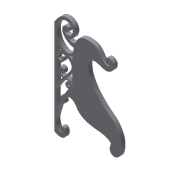
# Autodesk Inventor part: Sleigh
Saved by Autodesk Inventor 2014 (Build 180170000, 170)
## iProperties
Created: 2014-01-28
Part Number: Sleigh
Material: Generic
Document SubType Name: Modeling
Designer: caovt
Mass: 48.764 g
Surface Area: 236.408 cm^2
Volume: 48.764 cm^3
Density: 1 g/cm^3
Appearance: Default
Author: caovt
Autodesk Inventor part; units mm, degrees
ref_plane "YZ Plane" through (0, 0, 0) normal (1, 0, 0) x (0, 1, 0)
ref_plane "XZ Plane" through (0, 0, 0) normal (0, 1, 0) x (-1, 0, 0)
ref_plane "XY Plane" through (0, 0, 0) normal (0, 0, 1) x (1, 0, 0)
sketch "Sketch1" plane through (0, 0, 0) normal (0, 0, 1) x (1, 0, 0)
  line L0 (967.4531, 183.9202) -> (967.4531, 33.0728)
  spline S0 degree 3 poles (980.1584, 38.2097) (979.2094, 37.7398) (974.6095, 35.8122) (969.3206, 48.219) (972.1399, 59.141) (975.5351, 69.5204) (977.8227, 77.8537) (984.6298, 79.0574) (983.9258, 81.946) (982.297, 85.2802) (986.5076, 90.2314) (993.3177, 92.7761) (1000.3157, 88.1645) (1003.8658, 81.0591) (1010.8105, 74.3848) (1021.2008, 70.3973) (1033.4171, 68.679) (1045.4902, 67.7484) (1054.0616, 64.514) (1057.2209, 61.3406) (1057.5744, 60.9562) knots 0.025524 0.025524 0.025524 0.025524 0.114884 0.466054 0.840739 1.201389 1.495653 1.592606 1.644017 1.721232 1.930635 2.110051 2.356406 2.592626 2.837452 3.208473 3.582484 3.954767 4.317768 4.365528 4.365528 4.365528 4.365528
  line L1 (980.1584, 38.2097) -> (979.2094, 37.7398) construction
  line L2 (979.2094, 37.7398) -> (974.6095, 35.8122) construction
  line L3 (974.6095, 35.8122) -> (969.3206, 48.219) construction
  line L4 (969.3206, 48.219) -> (972.1399, 59.141) construction
  line L5 (972.1399, 59.141) -> (975.5351, 69.5204) construction
  line L6 (975.5351, 69.5204) -> (977.8227, 77.8537) construction
  line L7 (977.8227, 77.8537) -> (984.6298, 79.0574) construction
  line L8 (984.6298, 79.0574) -> (983.9258, 81.946) construction
  line L9 (983.9258, 81.946) -> (982.297, 85.2802) construction
  line L10 (982.297, 85.2802) -> (986.5076, 90.2314) construction
  line L11 (986.5076, 90.2314) -> (993.3177, 92.7761) construction
  line L12 (993.3177, 92.7761) -> (1000.3157, 88.1645) construction
  line L13 (1000.3157, 88.1645) -> (1003.8658, 81.0591) construction
  line L14 (1003.8658, 81.0591) -> (1010.8105, 74.3848) construction
  line L15 (1010.8105, 74.3848) -> (1021.2008, 70.3973) construction
  line L16 (1021.2008, 70.3973) -> (1033.4171, 68.679) construction
  line L17 (1033.4171, 68.679) -> (1045.4902, 67.7484) construction
  line L18 (1045.4902, 67.7484) -> (1054.0616, 64.514) construction
  line L19 (1054.0616, 64.514) -> (1057.2209, 61.3406) construction
  line L20 (1057.2209, 61.3406) -> (1057.5744, 60.9562) construction
  spline S1 degree 3 poles (1057.5744, 60.9562) (1057.1865, 59.9625) (1056.1068, 57.053) (1054.6206, 51.6931) (1059.07, 44.1064) (1070.5332, 46.3963) (1074.2538, 58.2626) (1074.5433, 70.5439) (1070.0117, 83.2884) (1061.747, 94.3239) (1050.6479, 101.5938) (1041.3803, 110.5746) (1033.3343, 119.2174) (1026.5395, 129.772) (1022.1641, 139.9181) (1021.4877, 149.7236) (1021.6835, 158.9558) (1031.3123, 162.2754) (1040.4018, 159.7346) (1050.8279, 155.5732) (1060.7215, 161.3305) (1063.4475, 171.8122) (1055.779, 178.2444) (1048.5769, 175.2818) (1047.8641, 169.1272) (1052.0071, 166.6972) (1054.5276, 166.8943) (1055.6122, 167.0837) knots 0.122315 0.122315 0.122315 0.122315 0.219275 0.403153 0.612556 0.886993 1.237331 1.640465 2.006704 2.440342 2.868406 3.201698 3.611753 3.93609 4.344072 4.583599 4.856399 5.067251 5.389035 5.719508 6.02994 6.307196 6.566006 6.753848 6.896235 7.026873 7.125917 7.125917 7.125917 7.125917
  line L21 (1057.5744, 60.9562) -> (1057.1865, 59.9625) construction
  line L22 (1057.1865, 59.9625) -> (1056.1068, 57.053) construction
  line L23 (1056.1068, 57.053) -> (1054.6206, 51.6931) construction
  line L24 (1054.6206, 51.6931) -> (1059.07, 44.1064) construction
  line L25 (1059.07, 44.1064) -> (1070.5332, 46.3963) construction
  line L26 (1070.5332, 46.3963) -> (1074.2538, 58.2626) construction
  line L27 (1074.2538, 58.2626) -> (1074.5433, 70.5439) construction
  line L28 (1074.5433, 70.5439) -> (1070.0117, 83.2884) construction
  line L29 (1070.0117, 83.2884) -> (1061.747, 94.3239) construction
  line L30 (1061.747, 94.3239) -> (1050.6479, 101.5938) construction
  line L31 (1050.6479, 101.5938) -> (1041.3803, 110.5746) construction
  line L32 (1041.3803, 110.5746) -> (1033.3343, 119.2174) construction
  line L33 (1033.3343, 119.2174) -> (1026.5395, 129.772) construction
  line L34 (1026.5395, 129.772) -> (1022.1641, 139.9181) construction
  line L35 (1022.1641, 139.9181) -> (1021.4877, 149.7236) construction
  line L36 (1021.4877, 149.7236) -> (1021.6835, 158.9558) construction
  line L37 (1021.6835, 158.9558) -> (1031.3123, 162.2754) construction
  line L38 (1031.3123, 162.2754) -> (1040.4018, 159.7346) construction
  line L39 (1040.4018, 159.7346) -> (1050.8279, 155.5732) construction
  line L40 (1050.8279, 155.5732) -> (1060.7215, 161.3305) construction
  line L41 (1060.7215, 161.3305) -> (1063.4475, 171.8122) construction
  line L42 (1063.4475, 171.8122) -> (1055.779, 178.2444) construction
  line L43 (1055.779, 178.2444) -> (1048.5769, 175.2818) construction
  line L44 (1048.5769, 175.2818) -> (1047.8641, 169.1272) construction
  line L45 (1047.8641, 169.1272) -> (1052.0071, 166.6972) construction
  line L46 (1052.0071, 166.6972) -> (1054.5276, 166.8943) construction
  line L47 (1054.5276, 166.8943) -> (1055.6122, 167.0837) construction
  spline S2 degree 3 poles (1055.6122, 167.0837) (1054.9244, 166.3452) (1052.8114, 164.365) (1046.8824, 166.1923) (1041.4592, 172.5726) (1036.6859, 182.0221) (1025.1045, 185.2257) (1013.9293, 185.3007) (1003.7093, 179.4626) (1001.4142, 169.4836) (994.7218, 169.1163) (991.9549, 170.1903) (990.7929, 170.7417) knots 0.02212 0.02212 0.02212 0.02212 0.109143 0.279583 0.491065 0.883092 1.17387 1.523301 1.891052 2.155702 2.308042 2.425214 2.425214 2.425214 2.425214
  line L48 (1055.6122, 167.0837) -> (1054.9244, 166.3452) construction
  line L49 (1054.9244, 166.3452) -> (1052.8114, 164.365) construction
  line L50 (1052.8114, 164.365) -> (1046.8824, 166.1923) construction
  line L51 (1046.8824, 166.1923) -> (1041.4592, 172.5726) construction
  line L52 (1041.4592, 172.5726) -> (1036.6859, 182.0221) construction
  line L53 (1036.6859, 182.0221) -> (1025.1045, 185.2257) construction
  line L54 (1025.1045, 185.2257) -> (1013.9293, 185.3007) construction
  line L55 (1013.9293, 185.3007) -> (1003.7093, 179.4626) construction
  line L56 (1003.7093, 179.4626) -> (1001.4142, 169.4836) construction
  line L57 (1001.4142, 169.4836) -> (994.7218, 169.1163) construction
  line L58 (994.7218, 169.1163) -> (991.9549, 170.1903) construction
  line L59 (991.9549, 170.1903) -> (990.7929, 170.7417) construction
  spline S3 degree 3 poles (998.4632, 163.0678) (997.8697, 160.7091) (997.4688, 158.2969) (997.1401, 155.8777) knots 0 0 0 0 1 1 1 1
  line L60 (998.4632, 163.0678) -> (997.8697, 160.7091) construction
  line L61 (997.8697, 160.7091) -> (997.4688, 158.2969) construction
  line L62 (997.4688, 158.2969) -> (997.1401, 155.8777) construction
  spline S4 degree 3 poles (996.6306, 151.4467) (996.3819, 148.7471) (996.2486, 146.0362) (996.1784, 143.3201) knots 0 0 0 0 1 1 1 1
  line L63 (996.6306, 151.4467) -> (996.3819, 148.7471) construction
  line L64 (996.3819, 148.7471) -> (996.2486, 146.0362) construction
  line L65 (996.2486, 146.0362) -> (996.1784, 143.3201) construction
  spline S5 degree 3 poles (996.1201, 128.7832) (996.1385, 123.1002) (996.1672, 117.4237) (996.1995, 111.7496) knots 1.164452 1.164452 1.164452 1.164452 1.680306 1.680306 1.680306 1.680306
  line L66 (996.1201, 128.7832) -> (996.1385, 123.1002) construction
  line L67 (996.1385, 123.1002) -> (996.1672, 117.4237) construction
  line L68 (996.1672, 117.4237) -> (996.1995, 111.7496) construction
  spline S6 degree 3 poles (998.4632, 163.0678) (996.5391, 163.5293) (992.041, 164.7941) (985.5685, 168.5652) (980.0167, 174.7644) (979.3546, 182.442) (983.2779, 187.1226) (988.1706, 187.6016) (991.0656, 184.079) (989.9389, 180.0393) (986.246, 179.0814) (984.5822, 180.2789) (983.6726, 180.9336) knots 0.101506 0.101506 0.101506 0.101506 0.280729 0.526162 0.772074 1.014944 1.144929 1.294358 1.389613 1.516616 1.597371 1.694757 1.694757 1.694757 1.694757
  line L69 (998.4632, 163.0678) -> (996.5391, 163.5293) construction
  line L70 (996.5391, 163.5293) -> (992.041, 164.7941) construction
  line L71 (992.041, 164.7941) -> (985.5685, 168.5652) construction
  line L72 (985.5685, 168.5652) -> (980.0167, 174.7644) construction
  line L73 (980.0167, 174.7644) -> (979.3546, 182.442) construction
  line L74 (979.3546, 182.442) -> (983.2779, 187.1226) construction
  line L75 (983.2779, 187.1226) -> (988.1706, 187.6016) construction
  line L76 (988.1706, 187.6016) -> (991.0656, 184.079) construction
  line L77 (991.0656, 184.079) -> (989.9389, 180.0393) construction
  line L78 (989.9389, 180.0393) -> (986.246, 179.0814) construction
  line L79 (986.246, 179.0814) -> (984.5822, 180.2789) construction
  line L80 (984.5822, 180.2789) -> (983.6726, 180.9336) construction
  spline S7 degree 3 poles (983.6726, 180.9336) (983.6684, 180.9196) (983.196, 179.3727) (984.999, 175.9747) (990.6639, 175.4455) (995.8565, 179.3886) (997.707, 186.8186) (992.5947, 193.4543) (983.665, 195.4531) (975.7854, 189.7908) (971.4433, 180.7219) (971.3636, 170.2172) (974.7684, 160.2649) (980.525, 154.0364) (986.3065, 151.2127) (991.4169, 151.3406) (994.6876, 153.8556) (996.5732, 155.4058) (997.1401, 155.8777) knots 0 0 0 0 0.044566 0.144788 0.296694 0.49525 0.693088 0.925339 1.173655 1.449015 1.73156 2.064748 2.375867 2.668572 2.807865 2.951079 3.104753 3.171724 3.171724 3.171724 3.171724
  line L81 (983.6726, 180.9336) -> (983.6684, 180.9196) construction
  line L82 (983.6684, 180.9196) -> (983.196, 179.3727) construction
  line L83 (983.196, 179.3727) -> (984.999, 175.9747) construction
  line L84 (984.999, 175.9747) -> (990.6639, 175.4455) construction
  line L85 (990.6639, 175.4455) -> (995.8565, 179.3886) construction
  line L86 (995.8565, 179.3886) -> (997.707, 186.8186) construction
  line L87 (997.707, 186.8186) -> (992.5947, 193.4543) construction
  line L88 (992.5947, 193.4543) -> (983.665, 195.4531) construction
  line L89 (983.665, 195.4531) -> (975.7854, 189.7908) construction
  line L90 (975.7854, 189.7908) -> (971.4433, 180.7219) construction
  line L91 (971.4433, 180.7219) -> (971.3636, 170.2172) construction
  line L92 (971.3636, 170.2172) -> (974.7684, 160.2649) construction
  line L93 (974.7684, 160.2649) -> (980.525, 154.0364) construction
  line L94 (980.525, 154.0364) -> (986.3065, 151.2127) construction
  line L95 (986.3065, 151.2127) -> (991.4169, 151.3406) construction
  line L96 (991.4169, 151.3406) -> (994.6876, 153.8556) construction
  line L97 (994.6876, 153.8556) -> (996.5732, 155.4058) construction
  line L98 (996.5732, 155.4058) -> (997.1401, 155.8777) construction
  spline S8 degree 3 poles (990.7929, 170.7417) (991.4872, 171.1598) (994.4624, 173.0013) (1000.2103, 178.0675) (1002.0786, 189.1751) (995.2704, 197.9354) (985.42, 200.362) (976.8631, 196.3938) (971.7761, 189.9597) (968.7177, 185.9676) (967.4531, 183.9202) knots 0.032478 0.032478 0.032478 0.032478 0.106187 0.350418 0.709182 1.002324 1.274671 1.568765 1.800056 2.018715 2.018715 2.018715 2.018715
  line L99 (990.7929, 170.7417) -> (991.4872, 171.1598) construction
  line L100 (991.4872, 171.1598) -> (994.4624, 173.0013) construction
  line L101 (994.4624, 173.0013) -> (1000.2103, 178.0675) construction
  line L102 (1000.2103, 178.0675) -> (1002.0786, 189.1751) construction
  line L103 (1002.0786, 189.1751) -> (995.2704, 197.9354) construction
  line L104 (995.2704, 197.9354) -> (985.42, 200.362) construction
  line L105 (985.42, 200.362) -> (976.8631, 196.3938) construction
  line L106 (976.8631, 196.3938) -> (971.7761, 189.9597) construction
  line L107 (971.7761, 189.9597) -> (968.7177, 185.9676) construction
  line L108 (968.7177, 185.9676) -> (967.4531, 183.9202) construction
  spline S9 degree 3 poles (971.2896, 94.1463) (972.1205, 95.6231) (975.2965, 101.0214) (980.0227, 107.4771) (984.075, 112.284) (985.1701, 113.5926) knots 0.380901 0.380901 0.380901 0.380901 0.534941 0.950474 1.105438 1.105438 1.105438 1.105438
  line L109 (971.2896, 94.1463) -> (972.1205, 95.6231) construction
  line L110 (972.1205, 95.6231) -> (975.2965, 101.0214) construction
  line L111 (975.2965, 101.0214) -> (980.0227, 107.4771) construction
  line L112 (980.0227, 107.4771) -> (984.075, 112.284) construction
  line L113 (984.075, 112.284) -> (985.1701, 113.5926) construction
  spline S10 degree 3 poles (987.381, 116.2662) (987.9331, 116.9466) (991.1016, 120.9295) (993.9005, 125.1864) (996.1201, 128.7832) knots 0 0 0 0 0.172077 1 1 1 1
  line L114 (987.381, 116.2662) -> (987.9331, 116.9466) construction
  line L115 (987.9331, 116.9466) -> (991.1016, 120.9295) construction
  line L116 (991.1016, 120.9295) -> (993.9005, 125.1864) construction
  line L117 (993.9005, 125.1864) -> (996.1201, 128.7832) construction
  spline S11 degree 3 poles (994.6348, 131.6945) (993.6555, 130.0171) (990.7573, 125.3685) (986.5566, 120.3717) (983.6369, 116.86) (982.9842, 116.0762) knots 0.243025 0.243025 0.243025 0.243025 0.419501 0.741473 0.834111 0.834111 0.834111 0.834111
  line L118 (994.6348, 131.6945) -> (993.6555, 130.0171) construction
  line L119 (993.6555, 130.0171) -> (990.7573, 125.3685) construction
  line L120 (990.7573, 125.3685) -> (986.5566, 120.3717) construction
  line L121 (986.5566, 120.3717) -> (983.6369, 116.86) construction
  line L122 (983.6369, 116.86) -> (982.9842, 116.0762) construction
  spline S12 degree 3 poles (980.7277, 113.375) (979.7324, 112.1897) (976.7484, 108.6675) (973.6699, 105.2221) (971.6233, 102.9316) knots 0 0 0 0 0.335182 1 1 1 1
  line L123 (980.7277, 113.375) -> (979.7324, 112.1897) construction
  line L124 (979.7324, 112.1897) -> (976.7484, 108.6675) construction
  line L125 (976.7484, 108.6675) -> (973.6699, 105.2221) construction
  line L126 (973.6699, 105.2221) -> (971.6233, 102.9316) construction
  spline S13 degree 3 poles (994.6348, 131.6945) (994.9399, 133.8516) (995.2532, 137.2819) (992.2946, 142.0241) (987.954, 145.1692) (981.5094, 146.8832) (976.0749, 144.3559) (972.5571, 140.4882) (973.8154, 136.0776) (976.9981, 135.8034) (979.9468, 136.5043) (979.4432, 138.2939) (977.6323, 138.8997) (979.2075, 141.4333) (982.6646, 142.195) (982.5674, 137.2046) (980.4782, 134.4411) (977.3041, 131.5208) (974.2634, 133.2583) (972.5684, 134.2483) (971.7371, 134.5498) (971.5487, 134.612) knots 0.028757 0.028757 0.028757 0.028757 0.21886 0.334367 0.516665 0.698273 0.909525 1.030232 1.142508 1.234015 1.313366 1.338753 1.380147 1.453009 1.522596 1.642961 1.756376 1.87233 1.97303 2.03608 2.054212 2.054212 2.054212 2.054212
  line L127 (994.6348, 131.6945) -> (994.9399, 133.8516) construction
  line L128 (994.9399, 133.8516) -> (995.2532, 137.2819) construction
  line L129 (995.2532, 137.2819) -> (992.2946, 142.0241) construction
  line L130 (992.2946, 142.0241) -> (987.954, 145.1692) construction
  line L131 (987.954, 145.1692) -> (981.5094, 146.8832) construction
  line L132 (981.5094, 146.8832) -> (976.0749, 144.3559) construction
  line L133 (976.0749, 144.3559) -> (972.5571, 140.4882) construction
  line L134 (972.5571, 140.4882) -> (973.8154, 136.0776) construction
  line L135 (973.8154, 136.0776) -> (976.9981, 135.8034) construction
  line L136 (976.9981, 135.8034) -> (979.9468, 136.5043) construction
  line L137 (979.9468, 136.5043) -> (979.4432, 138.2939) construction
  line L138 (979.4432, 138.2939) -> (977.6323, 138.8997) construction
  line L139 (977.6323, 138.8997) -> (979.2075, 141.4333) construction
  line L140 (979.2075, 141.4333) -> (982.6646, 142.195) construction
  line L141 (982.6646, 142.195) -> (982.5674, 137.2046) construction
  line L142 (982.5674, 137.2046) -> (980.4782, 134.4411) construction
  line L143 (980.4782, 134.4411) -> (977.3041, 131.5208) construction
  line L144 (977.3041, 131.5208) -> (974.2634, 133.2583) construction
  line L145 (974.2634, 133.2583) -> (972.5684, 134.2483) construction
  line L146 (972.5684, 134.2483) -> (971.7371, 134.5498) construction
  line L147 (971.7371, 134.5498) -> (971.5487, 134.612) construction
  spline S14 degree 3 poles (980.7277, 113.375) (979.8223, 113.5544) (977.2696, 114.1801) (973.5073, 116.8712) (972.7943, 122.2556) (975.5535, 127.8998) (982.2305, 126.7875) (983.5216, 122.2261) (982.2746, 118.6612) (979.1416, 118.3789) (978.1893, 120.2567) (979.1509, 121.6686) (980.397, 121.7827) (980.9837, 122.595) (980.8336, 124.2749) (977.8513, 124.8339) (975.8251, 122.6635) (976.2867, 119.3741) (978.7387, 116.0308) (981.544, 115.9553) (982.9842, 116.0762) knots 0.037832 0.037832 0.037832 0.037832 0.121834 0.276678 0.41964 0.586297 0.763614 0.869864 0.985858 1.053012 1.099293 1.144023 1.183711 1.204958 1.227846 1.324339 1.387999 1.474114 1.602336 1.725813 1.725813 1.725813 1.725813
  line L148 (980.7277, 113.375) -> (979.8223, 113.5544) construction
  line L149 (979.8223, 113.5544) -> (977.2696, 114.1801) construction
  line L150 (977.2696, 114.1801) -> (973.5073, 116.8712) construction
  line L151 (973.5073, 116.8712) -> (972.7943, 122.2556) construction
  line L152 (972.7943, 122.2556) -> (975.5535, 127.8998) construction
  line L153 (975.5535, 127.8998) -> (982.2305, 126.7875) construction
  line L154 (982.2305, 126.7875) -> (983.5216, 122.2261) construction
  line L155 (983.5216, 122.2261) -> (982.2746, 118.6612) construction
  line L156 (982.2746, 118.6612) -> (979.1416, 118.3789) construction
  line L157 (979.1416, 118.3789) -> (978.1893, 120.2567) construction
  line L158 (978.1893, 120.2567) -> (979.1509, 121.6686) construction
  line L159 (979.1509, 121.6686) -> (980.397, 121.7827) construction
  line L160 (980.397, 121.7827) -> (980.9837, 122.595) construction
  line L161 (980.9837, 122.595) -> (980.8336, 124.2749) construction
  line L162 (980.8336, 124.2749) -> (977.8513, 124.8339) construction
  line L163 (977.8513, 124.8339) -> (975.8251, 122.6635) construction
  line L164 (975.8251, 122.6635) -> (976.2867, 119.3741) construction
  line L165 (976.2867, 119.3741) -> (978.7387, 116.0308) construction
  line L166 (978.7387, 116.0308) -> (981.544, 115.9553) construction
  line L167 (981.544, 115.9553) -> (982.9842, 116.0762) construction
  spline S15 degree 3 poles (987.381, 116.2662) (988.2938, 116.0737) (990.5361, 115.4961) (992.6131, 114.0995) (993.4815, 113.0209) knots 0 0 0 0 0.403429 1 1 1 1
  line L168 (987.381, 116.2662) -> (988.2938, 116.0737) construction
  line L169 (988.2938, 116.0737) -> (990.5361, 115.4961) construction
  line L170 (990.5361, 115.4961) -> (992.6131, 114.0995) construction
  line L171 (992.6131, 114.0995) -> (993.4815, 113.0209) construction
  spline S16 degree 3 poles (990.2489, 102.5557) (988.69, 102.4113) (985.5926, 103.3787) (984.4991, 107.4467) (985.7932, 110.9948) (988.9297, 111.2356) (989.857, 109.3453) (988.8768, 107.9463) (987.6293, 107.8487) (987.032, 107.0442) (987.1598, 105.3625) (990.1344, 104.7641) (992.1892, 106.9075) (991.7712, 110.2027) (989.3743, 113.5632) (986.5928, 113.6894) (985.1701, 113.5926) knots 0.630814 0.630814 0.630814 0.630814 0.763614 0.869864 0.985858 1.053012 1.099293 1.144023 1.183711 1.204958 1.227846 1.324339 1.387999 1.474114 1.602336 1.724321 1.724321 1.724321 1.724321
  line L172 (990.2489, 102.5557) -> (988.69, 102.4113) construction
  line L173 (988.69, 102.4113) -> (985.5926, 103.3787) construction
  line L174 (985.5926, 103.3787) -> (984.4991, 107.4467) construction
  line L175 (984.4991, 107.4467) -> (985.7932, 110.9948) construction
  line L176 (985.7932, 110.9948) -> (988.9297, 111.2356) construction
  line L177 (988.9297, 111.2356) -> (989.857, 109.3453) construction
  line L178 (989.857, 109.3453) -> (988.8768, 107.9463) construction
  line L179 (988.8768, 107.9463) -> (987.6293, 107.8487) construction
  line L180 (987.6293, 107.8487) -> (987.032, 107.0442) construction
  line L181 (987.032, 107.0442) -> (987.1598, 105.3625) construction
  line L182 (987.1598, 105.3625) -> (990.1344, 104.7641) construction
  line L183 (990.1344, 104.7641) -> (992.1892, 106.9075) construction
  line L184 (992.1892, 106.9075) -> (991.7712, 110.2027) construction
  line L185 (991.7712, 110.2027) -> (989.3743, 113.5632) construction
  line L186 (989.3743, 113.5632) -> (986.5928, 113.6894) construction
  line L187 (986.5928, 113.6894) -> (985.1701, 113.5926) construction
  spline S17 degree 3 poles (996.1995, 111.7496) (995.9998, 111.5478) (995.3898, 111.2751) (994.3424, 112.2858) (993.6658, 112.867) (993.4815, 113.0209) knots 0 0 0 0 0.291909 0.803239 1 1 1 1
  line L188 (996.1995, 111.7496) -> (995.9998, 111.5478) construction
  line L189 (995.9998, 111.5478) -> (995.3898, 111.2751) construction
  line L190 (995.3898, 111.2751) -> (994.3424, 112.2858) construction
  line L191 (994.3424, 112.2858) -> (993.6658, 112.867) construction
  line L192 (993.6658, 112.867) -> (993.4815, 113.0209) construction
  spline S18 degree 3 poles (971.0289, 70.1167) (971.7531, 71.8074) (973.4313, 75.0945) (976.6251, 78.4965) (977.1826, 82.0692) (976.4184, 83.8288) (975.1577, 85.9814) (980.1266, 87.3806) (983.7556, 91.6574) (986.7225, 97.8453) (989.325, 101.3396) (990.2489, 102.5557) knots 0.15136 0.15136 0.15136 0.15136 0.318038 0.487404 0.563903 0.625415 0.667728 0.755317 0.961871 1.219224 1.358285 1.358285 1.358285 1.358285
  line L193 (971.0289, 70.1167) -> (971.7531, 71.8074) construction
  line L194 (971.7531, 71.8074) -> (973.4313, 75.0945) construction
  line L195 (973.4313, 75.0945) -> (976.6251, 78.4965) construction
  line L196 (976.6251, 78.4965) -> (977.1826, 82.0692) construction
  line L197 (977.1826, 82.0692) -> (976.4184, 83.8288) construction
  line L198 (976.4184, 83.8288) -> (975.1577, 85.9814) construction
  line L199 (975.1577, 85.9814) -> (980.1266, 87.3806) construction
  line L200 (980.1266, 87.3806) -> (983.7556, 91.6574) construction
  line L201 (983.7556, 91.6574) -> (986.7225, 97.8453) construction
  line L202 (986.7225, 97.8453) -> (989.325, 101.3396) construction
  line L203 (989.325, 101.3396) -> (990.2489, 102.5557) construction
  spline S19 degree 3 poles (971.0289, 70.1167) (971.0671, 73.1628) (971.1647, 81.1726) (971.2452, 89.1825) (971.2896, 94.1463) knots 0.215445 0.215445 0.215445 0.215445 0.492218 0.943221 0.943221 0.943221 0.943221
  line L204 (971.0289, 70.1167) -> (971.0671, 73.1628) construction
  line L205 (971.0671, 73.1628) -> (971.1647, 81.1726) construction
  line L206 (971.1647, 81.1726) -> (971.2452, 89.1825) construction
  line L207 (971.2452, 89.1825) -> (971.2896, 94.1463) construction
  spline S20 degree 3 poles (971.5921, 145.4774) (971.6067, 149.462) (971.6199, 153.4465) (971.6324, 157.4311) knots 0 0 0 0 1 1 1 1
  line L208 (971.5921, 145.4774) -> (971.6067, 149.462) construction
  line L209 (971.6067, 149.462) -> (971.6199, 153.4465) construction
  line L210 (971.6199, 153.4465) -> (971.6324, 157.4311) construction
  spline S21 degree 3 poles (996.6306, 151.4467) (995.811, 150.7177) (993.8161, 149.2211) (991.3482, 148.5619) (989.9444, 148.1986) knots 0 0 0 0 0.4335 1 1 1 1
  line L211 (996.6306, 151.4467) -> (995.811, 150.7177) construction
  line L212 (995.811, 150.7177) -> (993.8161, 149.2211) construction
  line L213 (993.8161, 149.2211) -> (991.3482, 148.5619) construction
  line L214 (991.3482, 148.5619) -> (989.9444, 148.1986) construction
  spline S22 degree 3 poles (996.1784, 143.3201) (995.4338, 144.0997) (993.6173, 145.8821) (991.4374, 147.4442) (990.0372, 148.1527) (989.9444, 148.1986) knots 0 0 0 0 0.406869 0.960862 1 1 1 1
  line L215 (996.1784, 143.3201) -> (995.4338, 144.0997) construction
  line L216 (995.4338, 144.0997) -> (993.6173, 145.8821) construction
  line L217 (993.6173, 145.8821) -> (991.4374, 147.4442) construction
  line L218 (991.4374, 147.4442) -> (990.0372, 148.1527) construction
  line L219 (990.0372, 148.1527) -> (989.9444, 148.1986) construction
  spline S23 degree 3 poles (971.6324, 157.4311) (971.9417, 157.0761) (973.5916, 155.1317) (975.4922, 152.3716) (977.8407, 150.8917) (978.4685, 150.5394) knots 0 0 0 0 0.144309 0.77977 1 1 1 1
  line L220 (971.6324, 157.4311) -> (971.9417, 157.0761) construction
  line L221 (971.9417, 157.0761) -> (973.5916, 155.1317) construction
  line L222 (973.5916, 155.1317) -> (975.4922, 152.3716) construction
  line L223 (975.4922, 152.3716) -> (977.8407, 150.8917) construction
  line L224 (977.8407, 150.8917) -> (978.4685, 150.5394) construction
  spline S24 degree 3 poles (978.4685, 150.5394) (977.6135, 150.12) (973.8217, 148.0385) (972.8683, 146.8115) (971.7051, 145.5943) (971.5921, 145.4774) knots 0 0 0 0 0.246961 0.929031 1 1 1 1
  line L225 (978.4685, 150.5394) -> (977.6135, 150.12) construction
  line L226 (977.6135, 150.12) -> (973.8217, 148.0385) construction
  line L227 (973.8217, 148.0385) -> (972.8683, 146.8115) construction
  line L228 (972.8683, 146.8115) -> (971.7051, 145.5943) construction
  line L229 (971.7051, 145.5943) -> (971.5921, 145.4774) construction
  spline S25 degree 3 poles (967.4531, 33.0728) (967.9488, 32.7151) (970.4518, 31.0694) (975.72, 29.4329) (984.5203, 30.749) (986.2595, 39.1104) (983.9366, 45.967) (978.9677, 45.841) (976.1476, 43.2968) (976.3664, 39.1628) (978.8057, 38.5676) (979.9712, 38.2596) (980.1584, 38.2097) knots 0.172484 0.172484 0.172484 0.172484 0.228419 0.447526 0.667275 0.932615 1.117298 1.210588 1.333691 1.427669 1.516771 1.534094 1.534094 1.534094 1.534094
  line L230 (967.4531, 33.0728) -> (967.9488, 32.7151) construction
  line L231 (967.9488, 32.7151) -> (970.4518, 31.0694) construction
  line L232 (970.4518, 31.0694) -> (975.72, 29.4329) construction
  line L233 (975.72, 29.4329) -> (984.5203, 30.749) construction
  line L234 (984.5203, 30.749) -> (986.2595, 39.1104) construction
  line L235 (986.2595, 39.1104) -> (983.9366, 45.967) construction
  line L236 (983.9366, 45.967) -> (978.9677, 45.841) construction
  line L237 (978.9677, 45.841) -> (976.1476, 43.2968) construction
  line L238 (976.1476, 43.2968) -> (976.3664, 39.1628) construction
  line L239 (976.3664, 39.1628) -> (978.8057, 38.5676) construction
  line L240 (978.8057, 38.5676) -> (979.9712, 38.2596) construction
  line L241 (979.9712, 38.2596) -> (980.1584, 38.2097) construction
  line L242 (971.5487, 134.612) -> (971.6233, 102.9316)
  constraints: 4 end point, 78 other
extrude "Extrusion1" add sketch "Sketch1" along normal blind 6.35
body "Solid1"
